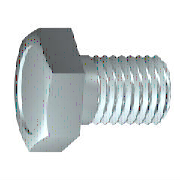
# Autodesk Inventor part: AS 1427 - M10 x 25
Saved by Autodesk Inventor 2021 (Build 250183000, 183)
## iProperties
Created: 2020-01-21
Part Number: AS 1427 - M10 x 25
Material: Steel, Mild
Description: ISO metric machine screws
Document SubType Name: Modeling
Standard: AS 1427
Designer: Angelos
Standards Organization: AS
Language: en-US
Size Designation: M10 x 25
Categories: <MemberInstance><Categories><Category DisplayName="Fasteners" InternalName="e4da775c-781d-43d5-af7c-5136215cf5a6" Mnemonic="FSTN"><Category DisplayName="Bolts" InternalName="536e6df0-f778-49ac-b2f2-25c71d2aa0b2" Mnemonic="SCRW"><CategoryParameter DisplayName="Nominal Diameter Designation" InternalName="03caf894-eafd-4c09-a035-916ac084b87b" Mnemonic="nomdiadesig"/><CategoryParameter DisplayName="Nominal Length" InternalName="238ecbaf-3e6c-45dd-aa95-4068c8e0fd02" Mnemonic="nomlen"/><CategoryParameter DisplayName="Thread Designation" InternalName="586d5e89-370a-4089-914f-0110033585c7" Mnemonic="thrdesign"/><CategoryParameter DisplayName="Thread Series Designation" InternalName="87c5849c-b3a5-4c3e-9c9b-2feecef9be86" Mnemonic="thrserdsgn"/><CategoryParameter DisplayName="Nominal Diameter" InternalName="8bbe3f8e-44cf-40a9-a251-3a6edc8168d6" Mnemonic="nomdia"/><CategoryParameter DisplayName="Thread Type" InternalName="b4bbb7bc-d6aa-4c9f-a9a9-4152b9f6fe49" Mnemonic="thrtype"/><CategoryParameter DisplayName="Thread Pitch" InternalName="bb82302e-82d8-4176-8fc1-c5d7bb17d5ad" Mnemonic="pitch1"/><CategoryParameter DisplayName="Threads per Unit" InternalName="bdc6e7d2-ffd0-4d9c-a173-16b95ebb912d" Mnemonic="thrperunit1"/><CategoryParameter DisplayName="Thread Class" InternalName="ebc0d23b-2cc6-4d2a-b376-d52aae53bab6" Mnemonic="thrclss"/><Category DisplayName="Hex Head" InternalName="520da9a1-ead7-4898-b571-59b4b339a5c6" Mnemonic="PLSCRW"><CategoryParameter DisplayName="Grip Length" InternalName="14b808f1-b175-4f80-b2c8-3c2ac1acde4c" Mnemonic="grplen"/><CategoryParameter DisplayName="Width Across Flats" InternalName="1cb53529-b7fd-49c5-a5c5-85a22d509c9e" Mnemonic="waflat"/><CategoryParameter DisplayName="Head Height" InternalName="3a45ce7b-b38d-4f77-aad7-a2328eea5aef" Mnemonic="headh"/><CategoryParameter DisplayName="Thread Length" InternalName="50b9771a-9fb7-48bc-803b-80099da79f2d" Mnemonic="thrlen"/><CategoryParameter DisplayName="Width Across Corners" InternalName="a21dc55e-7dbc-4faf-83dd-c7c1bfd07428" Mnemonic="wacor"/><CategoryParameter DisplayName="Shank Diameter" InternalName="bad16e07-a90c-44cc-a6af-8a6b56171876" Mnemonic="grpdia"/><CategoryParameter DisplayName="Diameter of Contact Area" InternalName="cc3b219b-8087-4820-96e9-69a08f47c1a6" Mnemonic="conardia"/></Category></Category></Category><Category DisplayName="DataType" InternalName="23b78d0f-2648-40c6-8793-ca6db495c9e8" Mnemonic="DATATYPE"><CategoryParameter DisplayName="DisplayName" InternalName="05415f3d-3907-474b-a020-eb9d644f4cf3" Mnemonic="DISPLAYNAME"/><CategoryParameter DisplayName="Standard" InternalName="0c0a119c-1e12-4c84-803f-101930972f5e" Mnemonic="STANDARD"/><CategoryParameter DisplayName="Description" InternalName="13903e3d-64b1-4950-80da-f627842ea37f" Mnemonic="DESCRIPTION"/><CategoryParameter DisplayName="Designation" InternalName="2675968c-4ce5-49e0-a4f5-552d29089031" Mnemonic="DESIGNATION"/><CategoryParameter DisplayName="Default Row" InternalName="2af9ec52-faaa-4026-b378-f9fa4afca842" Mnemonic="DEFAULTROW"/><CategoryParameter DisplayName="Folder Name" InternalName="3f06958e-8713-4116-9be7-ed6184ecc97b" Mnemonic="FOLDERNAME"/><CategoryParameter DisplayName="Revision Guid" InternalName="45a75005-10b1-4dfc-8d6d-dfe629f0b93c" Mnemonic="REVISIONGUID"/><CategoryParameter DisplayName="FileName" InternalName="8b46a4cc-9585-4fed-90c3-899f57e09a73" Mnemonic="FILENAME"/><CategoryParameter DisplayName="StdsOrg" InternalName="8f5914e1-4693-403f-8ab5-d37768198c9d" Mnemonic="STDSORG"/><CategoryParameter DisplayName="Family Version" InternalName="914462f6-6e19-4b14-ba84-155b9680b1d0" Mnemonic="FAMILYREVISION"/><CategoryParameter DisplayName="Standard Revision" InternalName="91d5a463-65c2-4fde-b823-3b7fea5e8e17" Mnemonic="STANDARDREVISION"/><CategoryParameter DisplayName="Member Revision" InternalName="a65d44b9-392f-4f4f-857b-e4b3d54996fe" Mnemonic="MEMBERREVISION"/><CategoryParameter DisplayName="ClipFormat" InternalName="bc51e27b-3422-4e78-93ef-cec197ddf230" Mnemonic="CLIPFORMAT"/><CategoryParameter DisplayName="Manufacturer" InternalName="cd6c7a72-a28a-4e50-99a9-2c7f4e13e5ad" Mnemonic="MANUFACTURER"/><CategoryParameter DisplayName="InternalName" InternalName="cf1d0246-76d9-4b4a-8305-fa0409afb5c1" Mnemonic="INTERNALNAME"/><CategoryParameter DisplayName="IsMetric" InternalName="e2385c5b-1ea4-4823-96a8-8de651266ec3" Mnemonic="ISMETRIC"/><Category DisplayName="Part" InternalName="c0e0b642-3bcb-4cc8-9e80-f96d35c4afa4" Mnemonic="PART"><CategoryParameter DisplayName="Part Number" InternalName="016b6077-bfbe-49bd-92c9-d8d59c39c941" Mnemonic="PARTNUMBER"/><CategoryParameter DisplayName="Stock Number" InternalName="4dba7c1c-e26c-444e-836c-b08b433409a8" Mnemonic="STOCKNUMBER"/><CategoryParameter DisplayName="Material Key" InternalName="5c9a8adb-dd2b-4535-b97f-0a94a95fe41f" Mnemonic="MATERIALKEY"/><CategoryParameter DisplayName="Material" InternalName="818a152a-d3c3-49ca-80ee-df7d91421b8e" Mnemonic="MATERIAL"/></Category></Category><Category DisplayName="LegacyMap" InternalName="cd87c42b-3e48-431e-b5c0-1cbeb14dfe77" Mnemonic="LEGACYMAP"><CategoryParameter DisplayName="unique DA member ID" InternalName="0918ad47-427f-4fed-ae26-24c81c58f590" Mnemonic="DACOOKIE"/><CategoryParameter DisplayName="Merge11 ID" InternalName="0ee8fb18-e2ed-4f39-96f6-1f4b5f50aa71" Mnemonic="MERGE11"/><CategoryParameter DisplayName="unique CC member ID" InternalName="5193edd4-b2b0-4ab4-9d54-de900eee34e0" Mnemonic="CCCOOKIE"/><CategoryParameter DisplayName="Split ID" InternalName="72b5c83c-be7f-45c4-ae51-9160ea6deb26" Mnemonic="SPLIT"/><CategoryParameter DisplayName="MemberID" InternalName="8e5e0294-fc51-4c8f-b3d7-003dc5ed94f6" Mnemonic="MEMBERID"/><CategoryParameter DisplayName="CatalogName" InternalName="d99d1e27-aa94-4de2-af4c-c348882a6f4f" Mnemonic="CATALOGNAME"/><CategoryParameter DisplayName="FamilyNumber" InternalName="e705e1f4-09cb-413e-91f9-551b4188271e" Mnemonic="FAMILYNUMBER"/></Category></Categories><FamilyTemplate Id="no0081"><FamilyTemplateParameters><FamilyTemplateParameter ObjectType="kUserParameterObject" ValueType="xs:double" Id="1" ObjectReferenceKey="GUL"/><FamilyTemplateParameter ObjectType="kUserParameterObject" ValueType="xs:double" Id="2" ObjectReferenceKey="SPD"/><FamilyTemplateParameter ObjectType="kUserParameterObject" ValueType="xs:double" Id="3" ObjectReferenceKey="NLG"/><FamilyTemplateParameter ObjectType="kUserParameterObject" ValueType="xs:double" Id="4" ObjectReferenceKey="TPU"/><FamilyTemplateParameter ObjectType="kUserParameterObject" ValueType="xs:double" Id="5" ObjectReferenceKey="GD1"/><FamilyTemplateParameter ObjectType="kUserParameterObject" ValueType="xs:double" Id="6" ObjectReferenceKey="GEL"/><FamilyTemplateParameter ObjectType="kUserParameterObject" ValueType="xs:double" Id="7" ObjectReferenceKey="SW"/><FamilyTemplateParameter ObjectType="kUserParameterObject" ValueType="xs:double" Id="8" ObjectReferenceKey="THREADDIA"/><FamilyTemplateParameter ObjectType="kUserParameterObject" ValueType="xs:double" Id="9" ObjectReferenceKey="SDH"/><FamilyTemplateParameter ObjectType="kUserParameterObject" ValueType="xs:double" Id="10" ObjectReferenceKey="ANG1"/><FamilyTemplateParameter ObjectType="kUserParameterObject" ValueType="xs:double" Id="11" ObjectReferenceKey="TOA"/><FamilyTemplateParameter ObjectType="kUserParameterObject" ValueType="xs:double" Id="12" ObjectReferenceKey="BDM"/><FamilyTemplateParameter ObjectType="kUserParameterObject" ValueType="xs:double" Id="13" ObjectReferenceKey="FAWI"/><FamilyTemplateParameter ObjectType="kUserParameterObject" ValueType="xs:double" Id="14" ObjectReferenceKey="RR"/><FamilyTemplateParameter ObjectType="kUserParameterObject" ValueType="xs:double" Id="15" ObjectReferenceKey="KOH"/><FamilyTemplateParameter ObjectType="kUserParameterObject" ValueType="xs:double" Id="16" ObjectReferenceKey="SW0"/><FamilyTemplateParameter ObjectType="kUserParameterObject" ValueType="xs:double" Id="17" ObjectReferenceKey="PTC"/><FamilyTemplateParameter ObjectType="kUserParameterObject" ValueType="xs:double" Id="18" ObjectReferenceKey="NND"/><FamilyTemplateParameter ObjectType="kUserParameterObject" ValueType="xs:double" Id="19" ObjectReferenceKey="GD"/><FamilyTemplateParameter ObjectType="kUserParameterObject" ValueType="xs:double" Id="20" ObjectReferenceKey="GAL"/><FamilyTemplateParameter ObjectType="kUserParameterObject" ValueType="xs:double" Id="21" ObjectReferenceKey="SD"/><FamilyTemplateParameter ObjectType="kUserParameterObject" ValueType="xs:double" Id="22" ObjectReferenceKey="SD2"/><FamilyTemplateParameter ObjectType="kUserParameterObject" ValueType="xs:double" Id="23" ObjectReferenceKey="E0"/><FamilyTemplateParameter ObjectType="kPropertyObject" ValueType="xs:string" Id="100" ObjectReferenceKey="{32853F0F-3444-11d1-9E93-0060B03C1CA6}" SubObjectId="52"/><FamilyTemplateParameter ObjectType="kPropertyObject" ValueType="xs:string" Id="105" ObjectReferenceKey="{32853F0F-3444-11d1-9E93-0060B03C1CA6}" SubObjectId="5"/><FamilyTemplateParameter ObjectType="kPartComponentDefinitionObject" ValueType="xs:string" Id="110" SubObjectId="Material"/><FamilyTemplateParameter ObjectType="kThreadFeatureObject" ValueType="xs:structure" Id="300" ObjectReferenceKey="100200001000000069050000000000008000000000000000" SubObjectId="ThreadInfo"><FamilyTemplateParameter ObjectType="" ValueType="xs:string" Id="301" SubObjectId="ThreadDesignation"/><FamilyTemplateParameter ObjectType="" ValueType="xs:string" Id="302" SubObjectId="ThreadType"/><FamilyTemplateParameter ObjectType="" ValueType="xs:string" Id="303" SubObjectId="ThreadClass"/></FamilyTemplateParameter></FamilyTemplateParameters></FamilyTemplate><CategoryParameterMap><ParamToTemplateMap><ParamToTemplate CategoryParameter="//CategoryParameter[@InternalName='05415f3d-3907-474b-a020-eb9d644f4cf3']" ConstantValue="AS 1427 - Metric"/><ParamToTemplate CategoryParameter="//CategoryParameter[@InternalName='cf1d0246-76d9-4b4a-8305-fa0409afb5c1']" ConstantValue="73bdd36a-873d-4dd6-8ae0-ce47c3b9e9c2"/><ParamToTemplate CategoryParameter="//CategoryParameter[@InternalName='3f06958e-8713-4116-9be7-ed6184ecc97b']" ConstantValue="AS 1427(02)"/><ParamToTemplate CategoryParameter="//CategoryParameter[@InternalName='914462f6-6e19-4b14-ba84-155b9680b1d0']" ConstantValue="10"/><ParamToTemplate CategoryParameter="//CategoryParameter[@InternalName='bc51e27b-3422-4e78-93ef-cec197ddf230']" ConstantValue="CF_INVENTOR.STDPARTS"/><ParamToTemplate CategoryParameter="//CategoryParameter[@InternalName='e2385c5b-1ea4-4823-96a8-8de651266ec3']" ConstantValue="true"/><ParamToTemplate CategoryParameter="//CategoryParameter[@InternalName='13903e3d-64b1-4950-80da-f627842ea37f']" ConstantValue="ISO metric machine screws"/><ParamToTemplate CategoryParameter="//CategoryParameter[@InternalName='8f5914e1-4693-403f-8ab5-d37768198c9d']" ConstantValue="AS"/><ParamToTemplate CategoryParameter="//CategoryParameter[@InternalName='0c0a119c-1e12-4c84-803f-101930972f5e']" ConstantValue="AS 1427"/><ParamToTemplate CategoryParameter="//CategoryParameter[@InternalName='cd6c7a72-a28a-4e50-99a9-2c7f4e13e5ad']" TemplateParameter="104"/><ParamToTemplate CategoryParameter="//CategoryParameter[@InternalName='91d5a463-65c2-4fde-b823-3b7fea5e8e17']" TemplateParameter="103"/><ParamToTemplate CategoryParameter="//CategoryParameter[@InternalName='45a75005-10b1-4dfc-8d6d-dfe629f0b93c']" ConstantValue="428ad986-a7c6-4a38-9275-8cd933b5f541"/><ParamToTemplate CategoryParameter="//CategoryParameter[@InternalName='2af9ec52-faaa-4026-b378-f9fa4afca842']" ConstantValue="10"/><ParamToTemplate CategoryParameter="//CategoryParameter[@InternalName='d99d1e27-aa94-4de2-af4c-c348882a6f4f']" ConstantValue="AS"/><ParamToTemplate CategoryParameter="//CategoryParameter[@InternalName='e705e1f4-09cb-413e-91f9-551b4188271e']" ConstantValue="13"/><ParamToTemplate CategoryParameter="//CategoryParameter[@InternalName='8b46a4cc-9585-4fed-90c3-899f57e09a73']" ConstantValue="AS 1427 - M10 x 25(2)"/><ParamToTemplate CategoryParameter="//CategoryParameter[@InternalName='a65d44b9-392f-4f4f-857b-e4b3d54996fe']" ConstantValue="D3E3584B-0760-4AFA-A0F1-EC4965BB2270"/><ParamToTemplate CategoryParameter="//CategoryParameter[@InternalName='14b808f1-b175-4f80-b2c8-3c2ac1acde4c']" ConstantValue="3"/><ParamToTemplate CategoryParameter="//CategoryParameter[@InternalName='ebc0d23b-2cc6-4d2a-b376-d52aae53bab6']" ConstantValue="6g"/><ParamToTemplate CategoryParameter="//CategoryParameter[@InternalName='03caf894-eafd-4c09-a035-916ac084b87b']" ConstantValue="M10"/><ParamToTemplate CategoryParameter="//CategoryParameter[@InternalName='b4bbb7bc-d6aa-4c9f-a9a9-4152b9f6fe49']" ConstantValue="ISO Metric profile"/><ParamToTemplate CategoryParameter="//CategoryParameter[@InternalName='8e5e0294-fc51-4c8f-b3d7-003dc5ed94f6']" ConstantValue="540"/><ParamToTemplate CategoryParameter="//CategoryParameter[@InternalName='bad16e07-a90c-44cc-a6af-8a6b56171876']" TemplateParameter="12"/><ParamToTemplate CategoryParameter="//CategoryParameter[@InternalName='2675968c-4ce5-49e0-a4f5-552d29089031']" TemplateParameter="100"/><ParamToTemplate CategoryParameter="//CategoryParameter[@InternalName='a21dc55e-7dbc-4faf-83dd-c7c1bfd07428']" TemplateParameter="23"/><ParamToTemplate CategoryParameter="//CategoryParameter[@InternalName='50b9771a-9fb7-48bc-803b-80099da79f2d']" TemplateParameter="6"/><ParamToTemplate CategoryParameter="//CategoryParameter[@InternalName='3a45ce7b-b38d-4f77-aad7-a2328eea5aef']" TemplateParameter="15"/><ParamToTemplate CategoryParameter="//CategoryParameter[@InternalName='818a152a-d3c3-49ca-80ee-df7d91421b8e']" TemplateParameter="110"/><ParamToTemplate CategoryParameter="//CategoryParameter[@InternalName='238ecbaf-3e6c-45dd-aa95-4068c8e0fd02']" TemplateParameter="3"/><ParamToTemplate CategoryParameter="//CategoryParameter[@InternalName='8bbe3f8e-44cf-40a9-a251-3a6edc8168d6']" TemplateParameter="18"/><ParamToTemplate CategoryParameter="//CategoryParameter[@InternalName='016b6077-bfbe-49bd-92c9-d8d59c39c941']" TemplateParameter="105"/><ParamToTemplate CategoryParameter="//CategoryParameter[@InternalName='bb82302e-82d8-4176-8fc1-c5d7bb17d5ad']" TemplateParameter="17"/><ParamToTemplate CategoryParameter="//CategoryParameter[@InternalName='586d5e89-370a-4089-914f-0110033585c7']" TemplateParameter="301"/><ParamToTemplate CategoryParameter="//CategoryParameter[@InternalName='bdc6e7d2-ffd0-4d9c-a173-16b95ebb912d']" TemplateParameter="4"/></ParamToTemplateMap></CategoryParameterMap></MemberInstance>
Density: 7.85 g/cm^3
Appearance: Semi-Polished
IsCustomPart: 0
Author: Angelos
Autodesk Inventor part; units mm, degrees
ref_plane "YZ Plane" through (0, 0, 0) normal (1, 0, 0) x (0, 1, 0)
ref_plane "XZ Plane" through (0, 0, 0) normal (0, 1, 0) x (-1, 0, 0)
sketch "Sketch1" plane through (0, 0, 0) normal (0, 0, 1) x (1, 0, 0)
  line L0 (0, 5) -> (0, 0)
  line L1 (0, 0) -> (25, 0)
  line L2 (25, 0) -> (25, 5)
  line L3 (25, 5) -> (0, 5)
  line L4 (-5, 0) -> (30, 0) projected
  line L5 (0, -1) -> (0, 6) projected
  dimension "d0" = 10
  dimension "d1" = 25
  constraints: 8 end point, 2 collinear, 2 parallel, 1 perpendicular, 1 point on line, 1 vertical
  measures "d0" diameter of L3 L1
  measures "d1" distance between parallel lines of L2 L0
revolve "Body" add sketch "Sketch1" angle 360 about axis through (0, 0, 0) along (1, 0, 0)
sketch "Sketch2" plane through (0, 0, 0) normal (1, 0, 0) x (0, 1, 0)
  line L0 (0, 9.815) -> (8.5, 4.9075)
  line L1 (8.5, 4.9075) -> (8.5, -4.9075)
  line L2 (8.5, -4.9075) -> (0, -9.815)
  line L3 (0, -9.815) -> (-8.5, -4.9075)
  line L4 (-8.5, -4.9075) -> (-8.5, 4.9075)
  line L5 (-8.5, 4.9075) -> (0, 9.815)
  line L6 (-11.9, 0) -> (11.9, 0) projected
  line L7 (0, -13.7409) -> (0, 13.7409) projected
  point P0 (0, 0)
  point P1 (0, 0)
  dimension "d2" = 17
  constraints: 12 end point, 2 midpoint, 1 coincident, 1 parallel, 11 other
  measures "d2" distance between parallel lines of L1 L4
extrude "Head" add sketch "Sketch2" against normal blind 8.23
sketch "Sketch3" plane through (-8.23, 0, 0) normal (-1, 0, 0) x (0, 1, 0)
  circle A0 centre (0, 0) radius 6.375
  point P0 (0, 0)
  dimension "d12" = 12.75
  constraints: 1 centre point, 1 coincident
  measures "d12" diameter of A0
extrude "Indent1" cut sketch "Sketch3" against normal blind 1.646
sketch "Sketch4" plane through (0, 0, 0) normal (0, 0, 1) x (1, 0, 0)
  line L0 (-8.23, 9.815) -> (-8.23, 8.5)
  line L1 (-8.23, 8.5) -> (-7.4708, 9.815)
  line L2 (-7.4708, 9.815) -> (-8.23, 9.815)
  line L3 (0, 9.815) -> (0, 8.5)
  line L4 (0, 8.5) -> (-0.7592, 9.815)
  line L5 (-0.7592, 9.815) -> (0, 9.815)
  line L6 (0, 0) -> (-8.23, 0) projected
  line L7 (-8.23, 0) -> (-8.23, 8.5) projected
  line L8 (0, 0) -> (0, 8.5) projected
  line L9 (-9.876, 0) -> (1.646, 0) projected
  line L10 (-7.4708, 9.815) -> (-0.7592, 9.815) construction
  line L11 (0, -1.963) -> (0, 11.7779) projected
  dimension "d6" = 30
  dimension "d7" = 30
  dimension "d16" = 17
  dimension "d17" = 17
  dimension "d18" = 19.6299
  constraints: 14 end point, 3 perpendicular, 2 collinear, 2 parallel, 1 vertical
  measures "d6" angle of L1 L0
  measures "d7" angle of L4 L3
  measures "d16" diameter of L0.end L9
  measures "d17" diameter of L3.end L9
  measures "d18" diameter of L2 L6
revolve "Chamfer1" cut sketch "Sketch4" angle 360 about axis through (-10, 0, 0) along (1, 0, 0)
fillet "Fillet1" radius 0.4 1 edges at (0, -5, 0)
thread "Thread" size "M10x1.5" class "6g" standard "ISO Metric profile" length 22
ref_plane "Work Plane1" through (3, 0, 0) normal (0, 0.5, 0.866) x (1, 0, 0)
equation "\"d0\" = GD"
equation "\"d1\" = NLG"
equation "\"d2\" = SW"
equation "\"d3\" = KOH"
equation "\"d12\" = 0.75 * SW0"
equation "\"d14\" = 0.2 * KOH"
equation "\"d6\" = ANG1"
equation "\"d7\" = ANG1"
equation "\"d16\" = SW0"
equation "\"d17\" = SW0"
equation "\"d18\" = 1.1547 * SW"
equation "\"d11\" = RR"
equation "\"d8\" = GEL"
equation "\"NLG\" = 25"
equation "\"KOH\" = 8.23"
equation "\"GD\" = NND"
equation "\"GEL\" = 22"
equation "\"SW\" = 17"
equation "\"SW0\" = SW"
equation "\"ANG1\" = 30deg"
equation "\"RR\" = 0.4"
equation "\"GUL\" = 0.61345 * PTC"
equation "\"SPD\" = NND - 1.2269 * PTC"
equation "\"GD1\" = THREADDIA - 1.2269 * PTC"
equation "\"SDH\" = 11.2"
equation "\"TOA\" = 30deg"
equation "\"FAWI\" = 45deg"
equation "\"PTC\" = 1.5"
equation "\"GAL\" = 0.61345 * PTC"
equation "\"SD\" = 0"
equation "\"SD2\" = SDH"
equation "\"E0\" = 1.155 * SW"
equation "\"NND\" = 10"
equation "\"THREADDIA\" = 10"
body "Solid1"
